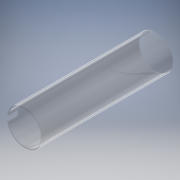
# Autodesk Inventor part: Crusher_Tube
Saved by Autodesk Inventor 2016 (Build 200138000, 138)
## iProperties
Created: 2016-04-23
Part Number: Crusher_Tube
Material: Generic
Document SubType Name: Modeling
Designer: 3DPrinterUser
Density: 1 g/cm^3
Appearance: Polycarbonate - Clear
Author: 3DPrinterUser
Autodesk Inventor part; units mm, degrees
ref_plane "YZ Plane" through (0, 0, 0) normal (1, 0, 0) x (0, 1, 0)
ref_plane "XZ Plane" through (0, 0, 0) normal (0, 1, 0) x (-1, 0, 0)
ref_plane "XY Plane" through (0, 0, 0) normal (0, 0, 1) x (1, 0, 0)
sketch "Sketch1" plane through (0, 0, 0) normal (0, 1, 0) x (-1, 0, 0)
  circle A0 centre (0, 0) radius 50
  circle A1 centre (0, 0) radius 53.5
  dimension "d0" = 100
  dimension "d1" = 3.5
  constraints: 2 centre point, 1 coincident
  measures "d0" diameter of A0
  measures "d1" radial gap between concentric circles of A0 A1
extrude "Extrusion1" add sketch "Sketch1" along normal blind 400
sketch "Sketch3" plane through (0, 0, 0) normal (1, 0, 0) x (0, 1, 0)
  spline S0 degree 3 poles (25, -8) (26.0064, -8) (27.0786, -7.7985) (29.0491, -6.9816) (29.9475, -6.3662) (31.3662, -4.9476) (31.9816, -4.0491) (32.7985, -2.0786) (33, -1.0063) (33, 1.0063) (32.7985, 2.0786) (31.9816, 4.0491) (31.3662, 4.9476) (29.9475, 6.3662) (29.0491, 6.9816) (27.0786, 7.7985) (26.0064, 8) (25, 8) knots -2.41526 -2.41526 -2.41526 -2.41526 -2.113349 -2.113349 -1.811438 -1.811438 -1.509534 -1.509534 -1.20763 -1.20763 -0.905726 -0.905726 -0.603822 -0.603822 -0.301911 -0.301911 0 0 0 0 projected
  line L0 (25, 8) -> (0, 8) projected
  line L1 (0, -8) -> (25, -8) projected
  line L2 (0, 8) -> (0, -8)
  line L3 (0, 53.5) -> (0, -53.5) projected
  point P0 (0, 0)
  constraints: 2 end point, 1 collinear
extrude "Extrusion2" cut sketch "Sketch3" against normal through all
body "Solid1"
